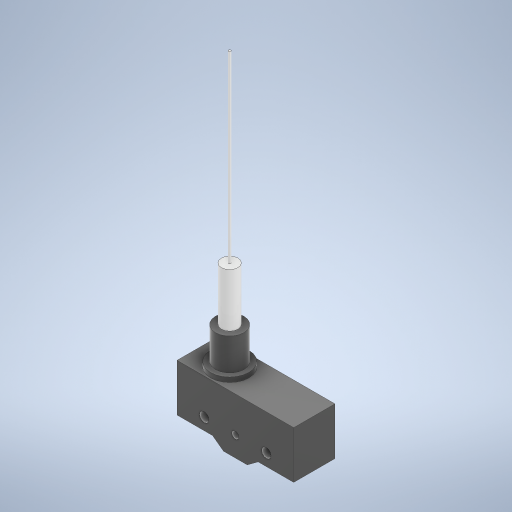
# Autodesk Inventor part: Z-15HNJS55-B
Saved by Autodesk Inventor 2023 (Build 270158000, 158)
## iProperties
Created: 2022-03-06
Part Number: Z-15HNJS55-B
Material: ABS プラスチック
Document SubType Name: Modeling
Designer: 中島 青蔵
Density: 1.06 g/cm^3
Appearance: 滑らか - 白
Author: 中島 青蔵
Autodesk Inventor part; units mm, degrees
ref_plane "YZ Plane" through (0, 0, 0) normal (1, 0, 0) x (0, 1, 0)
ref_plane "XZ Plane" through (0, 0, 0) normal (0, 1, 0) x (-1, 0, 0)
ref_plane "XY Plane" through (0, 0, 0) normal (0, 0, 1) x (1, 0, 0)
sketch "スケッチ1" plane through (0, 0, 0) normal (0, 0, 1) x (1, 0, 0)
  line L0 (0, 0) -> (49.2, 0)
  line L1 (49.2, 0) -> (49.2, 20)
  line L2 (49.2, 20) -> (0, 20)
  line L3 (0, 20) -> (0, 0)
  line L4 (15, 0) -> (19.5921, -3.4)
  line L5 (19.5921, -3.4) -> (29.6079, -3.4)
  line L6 (29.6079, -3.4) -> (34.2, 0)
  dimension "d0" = 49.2
  dimension "d1" = 20
  dimension "d2" = 15
  dimension "d3" = 15
  dimension "d4" = 3.4
  constraints: 14 end point, 2 parallel, 2 point on line, 1 equal length, 1 horizontal, 1 vertical
  measures "d0" distance of L2.end L1.end
  measures "d1" distance of L1.end L0.end
  measures "d2" distance of L0.start L4.start
  measures "d3" distance of L0.end L6.end
  measures "d4" distance between parallel lines of L0 L5
extrude "押し出し1" add sketch "スケッチ1" along normal blind 17.4
sketch "スケッチ2" plane through (0, 20, 0) normal (0, 1, 0) x (1, 0, 0)
  circle A0 centre (13.5, -8.7) radius 8.1
  line L0 (0, 0) -> (0, -17.4) projected
  circle A1 centre (13.5, -8.7) radius 6
  circle A2 centre (13.5, -8.7) radius 3.5
  dimension "d7" = 16.2
  dimension "d8" = 13.5
  dimension "d9" = 12
  dimension "d10" = 7
  constraints: 3 centre point, 2 coincident
  measures "d7" diameter of A0
  measures "d8" distance from line of L0 A0.centre
  measures "d9" diameter of A1
  measures "d10" diameter of A2
extrude "押し出し2" add sketch "スケッチ2" along normal blind 2 contours A0
extrude "押し出し3" add sketch "スケッチ2" along normal blind 15.5 contours A1
extrude "押し出し4" add sketch "スケッチ2" along normal blind 38 contours A2
sketch "スケッチ3" plane through (13.5, 58, 8.7) normal (0, 1, 0) x (1, 0, 0)
  circle A0 centre (0, 0) radius 0.5
  point P0 (-13.5, 8.7)
  dimension "d17" = 1
  constraints: 1 centre point
  measures "d17" diameter of A0
extrude "押し出し5" add sketch "スケッチ3" along normal blind 77.5
sketch "スケッチ4" plane through (0, 0, 17.4) normal (0, 0, 1) x (1, 0, 0)
  line L0 (0, 0) -> (15, 0) projected
  line L1 (34.2, 0) -> (49.2, 0) projected
  line L2 (49.2, 0) -> (49.2, 20) projected
  line L3 (0, 20) -> (0, 0) projected
  point P0 (11.5, 5)
  point P1 (37.7, 5)
  dimension "d20" = 5
  dimension "d21" = 5
  dimension "d22" = 11.5
  dimension "d23" = 11.5
  measures "d20" distance from line of L0 point (11.5, 5)
  measures "d21" distance from line of L1 point (37.7, 5)
  measures "d22" distance from line of L2 point (37.7, 5)
  measures "d23" distance from line of L3 point (11.5, 5)
hole "穴1" at (11.5, 5, 17.4) at (37.7, 5, 17.4) direction (0, 0, -1) diameter 4 end through all
sketch "スケッチ5" plane through (0, 0, 17.4) normal (0, 0, 1) x (1, 0, 0)
  circle A0 centre (11.5, 5) radius 2 projected
  circle A1 centre (37.7, 5) radius 2 projected
  line L0 (29.6079, -3.4) -> (34.2, 0) projected
  line L1 (34.2, 0) -> (49.2, 0) projected
  line L2 (49.2, 0) -> (49.2, 20) projected
  line L3 (49.2, 20) -> (0, 20) projected
  line L4 (0, 20) -> (0, 0) projected
  line L5 (0, 0) -> (15, 0) projected
  line L6 (15, 0) -> (19.5921, -3.4) projected
  line L7 (19.5921, -3.4) -> (29.6079, -3.4) projected
  circle A2 centre (24.6, 5) radius 1.5
  dimension "d31" = 3
  constraints: 1 centre point
  measures "d31" diameter of A2
extrude "押し出し6" cut sketch "スケッチ5" against normal blind 40 contours A2
